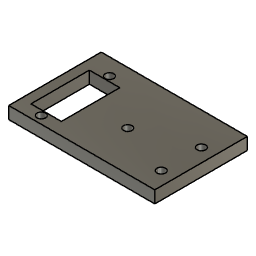
ServoBracket (Autodesk Fusion 360 design; units mm, degrees)
Autodesk Fusion 360 part; units mm, degrees
sketch "Sketch1" plane through (0, 0, 0) normal (0, 0, 1) x (1, 0, 0)
  line L0 (20.1643, 5) -> (80.1643, 5)
  line L1 (80.1643, 5) -> (80.1643, 43)
  line L2 (80.1643, 43) -> (20.1643, 43)
  line L3 (20.1643, 43) -> (20.1643, 5)
  line L4 (24.1483, 34.1483) -> (36.6483, 34.1483)
  line L5 (36.6483, 34.1483) -> (36.6483, 10.1483)
  line L6 (36.6483, 10.1483) -> (24.1483, 10.1483)
  line L7 (24.1483, 10.1483) -> (24.1483, 34.1483)
  circle A0 centre (74.6483, 29.6742) radius 1.75
  circle A1 centre (74.6483, 13.1742) radius 1.75
  line L8 (74.6483, 29.6742) -> (74.6483, 13.1742)
  line L9 (74.6483, 21.4242) -> (52.6483, 21.4242)
  circle A2 centre (52.6483, 21.4242) radius 1.75
  line L10 (95, 35) -> (105, 35)
  line L11 (105, 35) -> (105, 25)
  line L12 (105, 25) -> (95, 25)
  line L13 (95, 25) -> (95, 35)
  circle A3 centre (100, 30) radius 1.75
  circle A4 centre (30.3983, 8.1483) radius 1.75
  line L14 (24.1483, 22.1483) -> (9, 22.1483) construction
  circle A5 centre (30.3983, 36.1483) radius 1.75
  line L15 (80.1643, 27.7253) -> (80.1643, 24.8327)
  line L16 (36.6483, 24.8327) -> (36.6483, 27.7253)
  dimension "d1" = 60
  dimension "d2" = 38
  dimension "d3" = 24
  dimension "d4" = 12.5
  dimension "d6" = 3.5
  dimension "d7" = 16.5
  dimension "d8" = 3.5
  dimension "d9" = 38
  dimension "d10" = 22
  dimension "d11" = 3.5
  dimension "d12" = 3.5
  dimension "d16" = 3.5
  dimension "d17" = 2
  constraint horizontal L0
  constraint vertical L1
  constraint horizontal L2
  constraint vertical L3
  constraint horizontal L4
  constraint vertical L5
  constraint horizontal L6
  constraint vertical L7
  constraint coincident A0.centre L8.start
  constraint coincident A1.centre L8.end
  constraint parallel L1 L8
  constraint midpoint L8 L9.start
  constraint perpendicular L8 L9
  constraint coincident L9.end A2.centre
  constraint horizontal L10
  constraint vertical L11
  constraint horizontal L12
  constraint vertical L13
  constraint midpoint L7 L14.start
  constraint perpendicular L7 L14
  constraint symmetric A4 L14 A5
  constraint vertical L15
  constraint vertical L16
  constraint coincident L1 L15.end
  constraint coincident L5 L16.end
  measures "d1" distance of L1.end L2.end
  measures "d2" distance of L0.start L2.end
  measures "d3" distance of L4.start L6.end
  measures "d4" distance of L4.start L4.end
  measures "d6" diameter of A0
  measures "d7" distance of A0.centre A1.centre
  measures "d8" diameter of A1
  measures "d9" distance of L5 A0.centre
  measures "d10" distance of L9.start L9.end
  measures "d11" diameter of A2
  measures "d12" diameter of A3
  measures "d16" diameter of A4
  measures "d17" distance of L6 A4.centre
extrude "Extrude1" add sketch "Sketch1" along normal blind 5 contours L0 L1 L2 L3 L15 | L10 L11 L12 L13 | A4 | A5 makes body 1 at (41.3983, 21.907, 0) makes body 2 at (99.9564, 33.915, 0)
extrude "Extrude2" cut sketch "Sketch1" along normal blind 100 contours A4 | A5 bodies 1
delete_body "RemoveBody1" bodies 2
